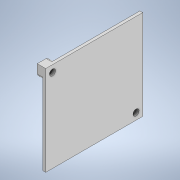
# Autodesk Inventor part: pokrywa_obudowa
Saved by Autodesk Inventor 2021 (Build 250183000, 183)
## iProperties
Created: 2025-11-29
Part Number: pokrywa_obudowa
Material: Generic
Document SubType Name: Modeling
Designer: huber
Density: 1 g/cm^3
Appearance: Default
Author: huber
Autodesk Inventor part; units mm, degrees
ref_plane "YZ Plane" through (0, 0, 0) normal (1, 0, 0) x (0, 1, 0)
ref_plane "XZ Plane" through (0, 0, 0) normal (0, 1, 0) x (-1, 0, 0)
ref_plane "XY Plane" through (0, 0, 0) normal (0, 0, 1) x (1, 0, 0)
sketch "Sketch1" plane through (0, 0, 0) normal (1, 0, 0) x (0, 1, 0)
  line L0 (32, 34.5) -> (-32, 34.5)
  line L1 (-32, 34.5) -> (-32, -34.5)
  line L2 (-32, -34.5) -> (32, -34.5)
  line L3 (32, -34.5) -> (32, 34.5)
  line L4 (32, 34.5) -> (-32, -34.5) construction
  line L5 (-32, 34.5) -> (32, -34.5) construction
  point P0 (0, 0)
  dimension "d0" = 69
  dimension "d1" = 64
  constraints: 12 end point, 2 midpoint, 2 parallel, 1 horizontal, 1 perpendicular
  measures "d0" distance between parallel lines of L2 L0
  measures "d1" distance of L1.end L2.end
extrude "Extrusion1" add sketch "Sketch1" along normal blind 2
sketch "Sketch2" plane through (0, 0, 0) normal (-1, 0, 0) x (0, 0, 1)
  circle A0 centre (29.5, 27) radius 3.75
  circle A1 centre (29.5, 27) radius 5
  line L0 (-34.5, 32) -> (34.5, 32) projected
  line L1 (34.5, 32) -> (34.5, -32) projected
  circle A2 centre (29.5, 27) radius 2.15
  point P0 (0, 0)
  point P1 (34.5, 27)
  point P2 (29.5, 32)
  dimension "d4" = 7.5
  dimension "d5" = 10
  dimension "d6" = 5
  dimension "d7" = 5
  dimension "d10" = 4.3
  constraints: 3 centre point, 2 coincident
  measures "d4" diameter of A0
  measures "d5" diameter of A1
  measures "d6" distance from line of L0 A0.centre
  measures "d7" distance from line of L1 A0.centre
  measures "d10" diameter of A2
extrude "Extrusion2" add sketch "Sketch2" along normal blind 4 contours A1 | A1 L0 L1
extrude "Extrusion3" cut sketch "Sketch2" against normal blind 4 contours A2
pattern_circular "Circular Pattern1" count 2 over 360 about axis through (-10, 0, 0) along (1, 0, 0) of "Extrusion2", "Extrusion3"
sketch "Sketch3" plane through (2, 0, 0) normal (1, 0, 0) x (0, 0, -1)
  circle A0 centre (29.5, -27) radius 2.15 projected
  circle A1 centre (-29.5, 27) radius 2.15 projected
  line L0 (-34.5, -32) -> (34.5, -32) projected
  line L1 (34.5, -32) -> (34.5, 32) projected
  line L2 (34.5, 32) -> (-34.5, 32) projected
  line L3 (-34.5, 32) -> (-34.5, -32) projected
  line L4 (-34.25, -31.75) -> (34.25, -31.75)
  line L5 (34.25, -31.75) -> (34.25, 31.75)
  line L6 (34.25, 31.75) -> (-34.25, 31.75)
  line L7 (-34.25, 31.75) -> (-34.25, -31.75)
  line L8 (-34.25, -31.75) -> (34.25, 31.75) construction
  line L9 (34.25, -31.75) -> (-34.25, 31.75) construction
  point P0 (0, 0)
  dimension "d16" = 0.25
  dimension "d17" = 0.25
  constraints: 12 end point, 2 midpoint, 2 parallel, 1 horizontal, 1 perpendicular
  measures "d16" distance between parallel lines of L2 L6
  measures "d17" distance between parallel lines of L3 L7
extrude "Extrusion4" cut sketch "Sketch3" against normal through all contours L3 L2 L1 L0
body "Solid1"
